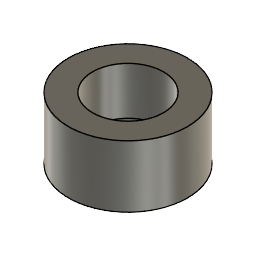
top rocket mount (Autodesk Fusion 360 design; units mm, degrees)
part number: 2026-02-07-17-15-43-592
Autodesk Fusion 360 part; units mm, degrees
sketch "Sketch1" plane through (0, 0, 0) normal (0, 0, 1) x (1, 0, 0)
  circle A0 centre (0, 0) radius 14.9
  circle A1 centre (0, 0) radius 25
  dimension "d32" = 50
  dimension "d44" = 29.8
  constraint coincident A0.centre A1.centre
  constraint concentric A0 A1
  measures "d32" diameter of A1
  measures "d44" diameter of A0
extrude "Extrude4" add sketch "Sketch1" along normal blind 6 contours A0
extrude "Extrude5" add sketch "Sketch1" along normal blind 26
